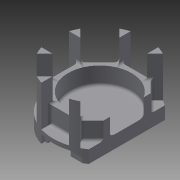
# Autodesk Inventor part: distance sensor mount
Saved by Autodesk Inventor 2015 (Build 190159000, 159)
## iProperties
Created: 2016-02-14
Part Number: distance sensor mount
Material: Generic
Document SubType Name: Modeling
Designer: -
Density: 1 g/cm^3
Appearance: Default
Author: -
Autodesk Inventor part; units mm, degrees
ref_plane "YZ Plane" through (0, 0, 0) normal (1, 0, 0) x (0, 1, 0)
ref_plane "XZ Plane" through (0, 0, 0) normal (0, 1, 0) x (-1, 0, 0)
ref_plane "XY Plane" through (0, 0, 0) normal (0, 0, 1) x (1, 0, 0)
sketch "Sketch7" plane through (0, 0, 0) normal (0, 1, 0) x (-1, 0, 0)
  circle A0 centre (0, 0) radius 26.556349
  circle A1 centre (0, 0) radius 23.556349
  circle A2 centre (0, 0) radius 34.556349
  line L0 (26.556349, 11) -> (26.556349, -11)
  line L1 (26.556349, -10.25) -> (33.001193, -10.25)
  line L2 (26.556349, 10.25) -> (33.001193, 10.25)
  line L3 (26.556349, 11) -> (11, 26.556349)
  line L4 (11, 26.556349) -> (-11, 26.556349)
  line L5 (-11, 26.556349) -> (-26.556349, 11)
  line L6 (-26.556349, 11) -> (-26.556349, -11)
  line L7 (-26.556349, -11) -> (-11, -26.556349)
  line L8 (-11, -26.556349) -> (11, -26.556349)
  line L9 (11, -26.556349) -> (26.556349, -11)
  line L10 (26.026019, 11.53033) -> (30.583212, 16.087523)
  line L11 (11.53033, 26.026019) -> (16.087523, 30.583212)
  line L12 (10.25, 26.556349) -> (10.25, 33.001193)
  line L13 (-10.25, 26.556349) -> (-10.25, 33.001193)
  line L14 (-26.026019, -11.53033) -> (-30.583212, -16.087523)
  line L15 (-11.53033, -26.026019) -> (-16.087523, -30.583212)
  line L16 (-10.25, -26.556349) -> (-10.25, -33.001193)
  line L17 (10.25, -26.556349) -> (10.25, -33.001193)
  line L18 (11.53033, -26.026019) -> (16.087523, -30.583212)
  line L19 (26.026019, -11.53033) -> (30.583212, -16.087523)
  line L20 (-26.556349, 10.25) -> (-33.001193, 10.25)
  line L21 (-26.556349, -10.25) -> (-33.001193, -10.25)
  line L22 (-26.026019, 11.53033) -> (-30.583212, 16.087523)
  line L23 (-11.53033, 26.026019) -> (-16.087523, 30.583212)
  line L24 (0, 0) -> (-13.224142, 31.925904)
  line L25 (-13.224142, -31.925904) -> (0, 0)
  line L26 (-20, 48.284271) -> (-20, -48.284271)
  point P0 (-20, 28.180512)
  point P1 (-20, -28.180512)
  point P2 (0, 26.556349)
  point P3 (18.778175, 18.778175)
  point P4 (26.556349, 0)
  point P5 (18.778175, -18.778175)
  point P6 (0, -26.556349)
  point P7 (-18.778175, -18.778175)
  point P8 (-20, -17.47111)
  point P9 (-20, -17.556349)
  point P10 (-20, -12.445947)
  point P11 (-20, 12.445947)
  point P12 (-20, 17.47111)
  point P13 (-20, 18.266998)
  point P14 (-18.778175, 18.778175)
  point P15 (-26.556349, 0)
  point P16 (-10.162675, 24.534867)
  point P17 (-9.014625, 21.763229)
  point P18 (-9.014625, -21.763229)
  point P19 (-10.162675, -24.534867)
  dimension "d67" = 8
  dimension "d66" = 3
  dimension "d69" = 135
  dimension "d70" = 22
  dimension "d71" = 0.75
  dimension "d72" = 0.75
  dimension "d73" = 0.75
  dimension "d74" = 0.75
  dimension "d75" = 0.75
  dimension "d76" = 0.75
  dimension "d77" = 0.75
  dimension "d78" = 0.75
  dimension "d79" = 0.75
  dimension "d80" = 0.75
  dimension "d81" = 0.75
  dimension "d82" = 0.75
  dimension "d83" = 0.75
  dimension "d84" = 0.75
  dimension "d85" = 0.75
  dimension "d86" = 0.75
  dimension "d87" = 20
  constraints: 52 end point, 25 point on line, 16 perpendicular, 8 midpoint, 7 equal length, 4 point on circle, 3 coincident, 3 vertical, 2 horizontal, 1 centre point, 50 other
  measures "d69" angle of L9 L0
  measures "d70" distance of L0.start L0.end
  measures "d71" distance from line of L2 L0.start
  measures "d72" distance from line of L0.end L1
  measures "d73" distance from line of L0.end L19
  measures "d74" distance from line of L17 L8.end
  measures "d75" distance from line of L7.end L16
  measures "d76" distance from line of L8.end L18
  measures "d77" distance from line of L7.end L15
  measures "d78" distance from line of L6.end L14
  measures "d79" distance from line of L6.end L21
  measures "d80" distance from line of L20 L5.end
  measures "d81" distance from line of L5.end L22
  measures "d82" distance from line of L4.end L23
  measures "d83" distance from line of L4.end L13
  measures "d84" distance from line of L3.end L12
  measures "d85" distance from line of L3.end L11
  measures "d86" distance from line of L0.start L10
sketch "Sketch8" plane through (0, 0, 0) normal (0, 1, 0) x (-1, 0, 0)
  line L0 (-8.5, 30) -> (-20, 30)
  line L1 (-20, 30) -> (-20, -30)
  line L2 (-20, -30) -> (-8.5, -30)
  line L3 (-8.5, -30) -> (-8.5, 30)
  line L4 (-20, 48.284271) -> (-20, -48.284271)
  circle A0 centre (0, 0) radius 34.556349
  line L5 (10.5, 32.922504) -> (10.5, 30)
  line L6 (10.5, 30) -> (8.5, 30)
  line L7 (8.5, 30) -> (8.5, -30)
  line L8 (8.5, -30) -> (10.5, -30)
  line L9 (10.5, -30) -> (10.5, -32.922504)
  point P0 (-20, 28.180512)
  point P1 (-17.150547, 30)
  point P2 (-17.150547, -30)
  point P3 (-20, -28.180512)
  dimension "d88" = 30
  dimension "d89" = 30
  dimension "d90" = 8.5
  dimension "d91" = 8.5
  dimension "d92" = 2
  constraints: 18 end point, 6 point on circle, 4 collinear, 4 point on line, 3 horizontal, 2 parallel, 2 vertical, 1 perpendicular
  measures "d88" distance from line of L2 point (0, 0)
  measures "d89" distance from line of L0 point (0, 0)
  measures "d90" distance from line of L3 point (0, 0)
  measures "d91" distance from line of L7 point (0, 0)
  measures "d92" distance between parallel lines of L7 L9
sketch "Sketch9" plane through (0, 0, 0) normal (0, 1, 0) x (-1, 0, 0)
  circle A0 centre (0, 0) radius 34.556349
  line L0 (-11.53033, 26.026019) -> (-16.087523, 30.583212)
  line L1 (-10.25, 26.556349) -> (-10.25, 33.001193)
  line L2 (10.25, 26.556349) -> (10.25, 33.001193)
  line L3 (11.53033, 26.026019) -> (16.087523, 30.583212)
  line L4 (26.026019, 11.53033) -> (30.583212, 16.087523)
  line L5 (26.556349, 10.25) -> (33.001193, 10.25)
  line L6 (26.556349, -10.25) -> (33.001193, -10.25)
  line L7 (26.026019, -11.53033) -> (30.583212, -16.087523)
  line L8 (11.53033, -26.026019) -> (16.087523, -30.583212)
  line L9 (10.25, -26.556349) -> (10.25, -33.001193)
  line L10 (-10.25, -26.556349) -> (-10.25, -33.001193)
  line L11 (-26.026019, -11.53033) -> (-30.583212, -16.087523)
  line L12 (-26.556349, -10.25) -> (-33.001193, -10.25)
  line L13 (-26.556349, 10.25) -> (-33.001193, 10.25)
  line L14 (-26.026019, 11.53033) -> (-30.583212, 16.087523)
  line L15 (-11.53033, -26.026019) -> (-16.087523, -30.583212)
  line L16 (11.53033, 26.026019) -> (10.25, 24.745689)
  line L17 (10.25, 24.745689) -> (10.25, 26.556349)
  line L18 (-11.53033, 26.026019) -> (-10.25, 24.745689)
  line L19 (-10.25, 24.745689) -> (-10.25, 26.556349)
  line L20 (-26.026019, 11.53033) -> (-24.745689, 10.25)
  line L21 (-24.745689, 10.25) -> (-26.556349, 10.25)
  line L22 (-26.556349, -10.25) -> (-24.745689, -10.25)
  line L23 (-24.745689, -10.25) -> (-26.026019, -11.53033)
  line L24 (-10.25, -24.745689) -> (-10.25, -26.556349)
  line L25 (10.25, -26.556349) -> (10.25, -24.745689)
  line L26 (10.25, -24.745689) -> (11.53033, -26.026019)
  line L27 (26.026019, -11.53033) -> (24.745689, -10.25)
  line L28 (24.745689, -10.25) -> (26.556349, -10.25)
  line L29 (26.556349, 10.25) -> (24.745689, 10.25)
  line L30 (26.026019, 11.53033) -> (24.745689, 10.25)
  line L31 (-10.25, -24.745689) -> (-11.53033, -26.026019)
  constraints: 32 end point, 16 collinear, 1 other
extrude "Extrusion9" add sketch "Sketch7" along normal blind 3 contours A0 L25 A1 L24 | L0 L9 A0 | A0 L3 L0 | L0 L2 A2 L1 | L3 L11 A2 L10 | A0 L4 L3 | L9 L8 A0 | L9 L19 A2 L18 | L0 L3 L10 A2 L2 | L1 A2 L19 L9 L0 | L4 L13 A2 L12 | A0 L24 L4 | L3 L4 L12 A2 L11 | L8 L25 A0 | L8 L17 A2 L16 | L18 A2 L17 L8 L9 | L24 A1 L26 A0 | A0 L5 L24 | L4 L24 A2 L13 | L25 L7 A0 | A0 L26 A1 L25 | L16 A2 L25 L8 | L5 L26 A2 L23 | A0 L26 L5 | L24 L25 A1 L26 | A1 L25 L24 | L5 L23 A2 L24 | L7 L15 A2 L26 | L25 A2 L15 L7
extrude "Extrusion10" add sketch "Sketch7" along normal blind 16 contours A0 L25 A1 L24 | L0 L9 A0 | A0 L3 L0 | A0 L4 L3 | L9 L8 A0 | L0 L3 L10 A2 L2 | L1 A2 L19 L9 L0 | A0 L24 L4 | L3 L4 L12 A2 L11 | L8 L25 A0 | L18 A2 L17 L8 L9 | L24 A1 L26 A0 | A0 L5 L24 | L4 L24 A2 L13 | L25 L7 A0 | A0 L26 A1 L25 | L16 A2 L25 L8 | L5 L23 A2 L24 | L7 L26 A0 | L25 A2 L15 L7
extrude "Extrusion11" add sketch "Sketch9" along normal blind 33 contours L5 L29 L30 L4 A0 | A0 L7 L27 L28 L6 | L3 L16 L17 L2 A0 | A0 L9 L25 L26 L8 | L1 L19 L18 L0 A0 | A0 L15 L31 L24 L10
extrude "Extrusion12" add sketch "Sketch8" against normal blind 6.4 contours L3 L2 A0 L1 L0 | A0 L9 L8 L7 L6 L5
chamfer "Chamfer4" distance 3 angle 45 4 edges at (12.8253, 0, 30) (12.8253, 0, -30) (-9.5, 0, -30) (-9.5, 0, 30)
chamfer "Chamfer5" distance 1.5 angle 45 6 edges at (-8.5, 0, 31.5) (-8.5, 0, 0) (-8.5, 0, -31.5) (8.5, 0, 31.5) (8.5, 0, -31.5) (8.5, 0, 0)
fillet "Fillet4" radius 2 19 edges at (15.7652, 3, -21.7912) (11.5303, 9.5, -26.026) (19.4001, 3, 18.1349) (15.1543, 3, 22.4021) (11.5303, 9.5, 26.026) (10.25, 9.5, 26.5563) (0, 3, 26.5563) (-18.7782, 3, 18.7782) (-26.026, 9.5, 11.5303) (-10.25, 9.5, 26.5563) (-26.5563, 9.5, -10.25) (-26.5563, 3, 0) (-26.5563, 9.5, 10.25) (-18.7782, 3, -18.7782) (-26.026, 9.5, -11.5303) (-11.5303, 9.5, -26.026) (-10.25, 9.5, -26.5563) (0, 3, -26.5563) (10.25, 9.5, -26.5563)
fillet "Fillet5" radius 2 1 edges at (-23.5563, 3, 0)
fillet "Fillet6" radius 2 23 edges at (10.25, 16, 25.651) (10.25, 16, 27.5563) (-10.8902, 16, 25.3859) (-25.651, 16, 10.25) (-27.5563, 16, 10.25) (-10.8902, 16, -25.3859) (-12.2374, 16, -26.7331) (10.25, 16, -25.651) (10.25, 16, -27.5563) (10.8902, 16, 25.3859) (12.2374, 16, 26.7331) (10.8902, 16, -25.3859) (12.2374, 16, -26.7331) (-10.25, 16, -25.651) (-10.25, 16, -27.5563) (-10.25, 16, 25.651) (-10.25, 16, 27.5563) (-25.3859, 16, 10.8902) (-26.7331, 16, 12.2374) (-25.3859, 16, -10.8902) (-26.7331, 16, -12.2374) (-25.651, 16, -10.25) (-27.5563, 16, -10.25)
body "Solid5"
